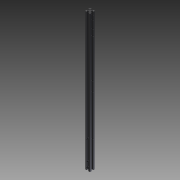
# Autodesk Inventor part: HFSB5-2020-550-LCH-RWV-AH30-BH60-CH85-DH240-EH280-AP442
Saved by Autodesk Inventor 2011 SP1 (Build 150282100, 282)
## iProperties
Created: 2016-03-22
Part Number: HFSB5-2020-550-LCH-RWV-AH30-BH60-CH85-DH240-EH280-AP442
Catalog Web Link: www.cadenas.de
Description: NFS5-2020, NFSB5-2020, HFS5-2020, HFSB5-2020, CAF5-2020, HFSY5-2020, NFSF5-2020, HFSF5-2020, HFSFB5-2020, NFST5-2020, HFST5-2020, HFSTB5-2020, HFSH5-2020, HFSC5-2020-HFS5 Series Aluminum Extrusions 20 Square -1 Slot-
Vendor: MISUMI
Document SubType Name: Modeling
Designer: psAdmin
Manufacturer: MISUMI
Mass: 97.771 g
Surface Area: 953.438 cm^2
Volume: 97.771 cm^3
Density: 1 g/cm^3
Category: PARTsolutions
Company: MISUMI
Title: HFSB5-2020-550-LCH-RWV-AH30-BH60-CH85-DH240-EH280-AP442
Author: Cadenas PARTsolutions
Comments: HFS5 Series Aluminum Extrusions 20 Square -1 Slot-
PSOL_IDENT_0: {$CADENAS_DATA\23d-libs\misumi\metric\38_al_extrusions_blackets\5\hfs5_2020.prj},654 {VTYP=3D},{NB=H
PSOL_IDENT_1: FSB5-2020-550-LCH-RWV-AH30-BH60-CH85-DH240-EH280-AP442},{LINA=HFSB5-2020-550-LCH-RWV-AH30-BH60-CH85-
PSOL_IDENT_2: DH240-EH280-AP442},{NN=NFS5-2020, NFSB5-2020, HFS5-2020, HFSB5-2020, CAF5-2020, HFSY5-2020, NFSF5-20
PSOL_IDENT_3: 20, HFSF5-2020, HFSFB5-2020, NFST5-2020, HFST5-2020, HFSTB5-2020, HFSH5-2020, HFSC5-2020},{DATE=17.0
PSOL_IDENT_4: 7.2015 10:47:07},{GEOMDATE=28.10.2014 00:00:00},{VERSION=},{LINEID=140},{LINESUBID=-1},{WBVAR=L,ALT1
PSOL_IDENT_5: ,ALT2,ALT4,ALT5,CP5,DL5,DR5,ALT6,ALT9,ALT10,ALT11,HP6,NHL6,DL6,NHR6,DR6,ALT7,ALT8,NH9,AH,BH,CH,DH,EH
PSOL_IDENT_6: ,NH10,AV,BV,CV,DV,EV,NH11,AP,BP,CP,DP,EP,ALT12,ALT13,Z,NH12,XA,XB,XC,XD,XE,NH13,YA,YB,YC,YD,YE,ALT16
PSOL_IDENT_7: ,HP16,DL16,DR16,ALT17,HQ17,JLP,ALT20}  {NB=HFSB5-2020-550-LCH-RWV-AH30-BH60-CH85-DH240-EH280-AP442},
PSOL_IDENT_8: {LINA=HFSB5-2020-550-LCH-RWV-AH30-BH60-CH85-DH240-EH280-AP442},{KT=DUMMY},{PN=HFSB5-2020-550-LCH-RWV
PSOL_IDENT_9: -AH30-BH60-CH85-DH240-EH280-AP442},{TPS=HFSB5-2020},{MAT=A6N01SS-T5 Aluminum Alloy or 6005A-T5 Alumi
PSOL_IDENT_10: num Alloy},{ST=Black Anodize},{FRMW=20},{FRMH=20},{FRD=4.2},{L=550},{MASS=0.5},{SA=183},{LX=0.742x10
PSOL_IDENT_11: ^4},{LY=0.742x10^4},{ALT1=},{M1=0},{DPL1=0},{DPR1=0},{ALT1PN=},{ALT2=},{ALT2ALG= '','w/o End Tapping
PSOL_IDENT_12: (Heli-Coil Insert)','LHP','with LHP (Tapping on the Left (Heli-Coil Insert))','RHP','with RHP (Tapp
PSOL_IDENT_13: ing on the Right (Heli-Coil Insert))','HPW','with HPW (Tapping on Both Ends (Heli-Coil Insert))' },{
PSOL_IDENT_14: M2=0},{DP2=0},{ALT2PN=},{ALT4=},{ALT4ALG= '', 'w/o SC (High Precision Cut)', 'SC', 'with SC (High Pr
PSOL_IDENT_15: ecision Cut)' },{ALT4PN=},{ALT5=},{ALT5ALG= '','w/o 45 Degree Cut','1','with 45 Degree Cut' },{CP5=}
PSOL_IDENT_16: ,{CP5ALG= '','N/A' },{DL5=},{DL5ALG= '','N/A' },{DR5=},{DR5ALG= '','N/A' },{FRMLALT5=0},{FRMRALT5=0}
PSOL_IDENT_17: ,{ALT5PN=},{ALT6=1},{ALT6ALG= '','w/o Fastening Location Wrench Access Hole Alterations','1','with F
PSOL_IDENT_18: astening Location Wrench Access Hole Alterations' },{ALT9=1},{ALT9ALG= '','w/o Location Specified Wr
PSOL_IDENT_19: ench Access Hole Alteratons (Horizontal)','1','with Location Specified Wrench Access Hole Alteratons
PSOL_IDENT_20: (Horizontal)' },{ALT10=},{ALT10ALG= '','w/o Location Specified Wrench Access Hole Alteratons (Verti
PSOL_IDENT_21: cal)','1','with Location Specified Wrench Access Hole Alteratons (Vertical)' },{ALT11=1},{ALT11ALG= ''
PSOL_IDENT_22: ,'w/o Location Specified Wrench Access Hole Alteratons (Crisscross)','1','with Location Specified Wr
PSOL_IDENT_23: ench Access Hole Alteratons (Crisscross)' },{HP6=LR},{HP6ALG= 'L','Left','R','Right','LR','Both Side
PSOL_IDENT_24: s' },{NHL6=C},{NHL6ALG= 'C','C (Wrench Holes in Single Line)','W','W (Wrench Holes in Two Lines)','E'
PSOL_IDENT_25: ,'E (Wrench Holes in Three Lines)' },{DL6=H},{DL6ALG= 'H','H (Horizontal)','V','V (Vertical)','P','P
PSOL_IDENT_26: (Crisscross)' },{NHR6=W},{NHR6ALG= 'C','C (Wrench Holes in Single Line)','W','W (Wrench Holes in Tw
PSOL_IDENT_27: o Lines)','E','E (Wrench Holes in Three Lines)' },{DR6=V},{DR6ALG= 'H','H (Horizontal)','V','V (Vert
PSOL_IDENT_28: ical)','P','P (Crisscross)' },{HL6=10},{HL6D=10},{HR6=10},{HR6D=10},{J6=20},{J6D=20},{K6=20},{K6D=0}
PSOL_IDENT_29: ,{DD6=7.35},{DD6ALG=7.35},{ALT7=},{ALT7ALG= '','w/o FL (Shifts The Wrench Hole on The Left Side 3mm
PSOL_IDENT_30: Toward The Left End)','FL','with FL (Shifts The Wrench Hole on The Left Side 3mm Toward The Left End
PSOL_IDENT_31: )' },{ALT8=},{ALT8ALG= '','w/o FR (Shifts The Wrench Hole on The Right Side 3mm Toward The Right End
PSOL_IDENT_32: )','FR','with FR (Shifts The Wrench Hole on The Right Side 3mm Toward The Right End)' },{ALT678PN=-L
PSOL_IDENT_33: CH-RWV},{NH9=5},{NH9MAX=5},{NH9ALG=[1:5/1]},{AH=30.0},{AHMIN=7},{AHMAX=505},{AHALG=[7:505/0.5]},{BH=
PSOL_IDENT_34: 60.0},{BHMIN=39.5},{BHMAX=514.5},{BHALG=[39.5:514.5/0.5]},{CH=85.0},{CHMIN=69.5},{CHMAX=524},{CHALG=
PSOL_IDENT_35: [69.5:524/0.5]},{DH=240.0},{DHMIN=94.5},{DHMAX=533.5},{DHALG=[94.5:533.5/0.5]},{EH=280.0},{EHMIN=249
PSOL_IDENT_36: .5},{EHMAX=543},{EHALG=[249.5:543/0.5]},{NH10=0},{NH10MAX=5},{NH10ALG=[0]},{AV=0.0},{AVMIN=7},{AVMAX=
PSOL_IDENT_37: 552.5},{AVALG=[0]},{BV=0.0},{BVMIN=9.5},{BVMAX=562},{BVALG=[0]},{CV=0.0},{CVMIN=9.5},{CVMAX=571.5},{
PSOL_IDENT_38: CVALG=[0]},{DV=0.0},{DVMIN=9.5},{DVMAX=581},{DVALG=[0]},{EV=0.0},{EVMIN=9.5},{EVMAX=543},{EVALG=[0]}
PSOL_IDENT_39: ,{NH11=1},{NH11MAX=5},{NH11ALG=[1:5/1]},{AP=442.0},{APMIN=7},{APMAX=543},{APALG=[7:543/0.5]},{BP=0.0
PSOL_IDENT_40: },{BPMIN=451.5},{BPMAX=552.5},{BPALG=[0]},{CP=0.0},{CPMIN=9.5},{CPMAX=562},{CPALG=[0]},{DP=0.0},{DPM
PSOL_IDENT_41: IN=9.5},{DPMAX=571.5},{DPALG=[0]},{EP=0.0},{EPMIN=9.5},{EPMAX=543},{EPALG=[0]},{ALT9PN=-AH30-BH60-CH
PSOL_IDENT_42: 85-DH240-EH280},{ALT10PN=},{ALT11PN=-AP442},{ALT91011PN=-AH30-BH60-CH85-DH240-EH280-AP442},{ALT12=},
PSOL_IDENT_43: {ALT12ALG= '','w/o Counterbore Hole in Specified Position (Vertical)','1','with Counterbore Hole in
PSOL_IDENT_44: Specified Position (Vertical)' },{ALT13=},{ALT13ALG= '','w/o Counterbore Hole in Specified Position
PSOL_IDENT_45: (Horizontal)','1','with Counterbore Hole in Specified Position (Horizontal)' },{Z=},{ZALG= '','N/A'
PSOL_IDENT_46: },{DD12=0.0},{DD112=0.0},{NH12=0},{NH12MAX=5},{NH12ALG=[0]},{XA=0.0},{XAMIN=7},{XAMAX=545},{XAALG=[0
PSOL_IDENT_47: ]},{XB=0.0},{XBMIN=2},{XBMAX=547},{XBALG=[0]},{XC=0.0},{XCMIN=2},{XCMAX=549},{XCALG=[0]},{XD=0.0},{X
PSOL_IDENT_48: DMIN=2},{XDMAX=551},{XDALG=[0]},{XE=0.0},{XEMIN=2},{XEMAX=543},{XEALG=[0]},{NH13=0},{NH13MAX=5},{NH1
PSOL_IDENT_49: 3ALG=[0]},{YA=0.0},{YAMIN=7},{YAMAX=545},{YAALG=[0]},{YB=0.0},{YBMIN=2},{YBMAX=547},{YBALG=[0]},{YC=
PSOL_IDENT_50: 0.0},{YCMIN=2},{YCMAX=549},{YCALG=[0]},{YD=0.0},{YDMIN=2},{YDMAX=551},{YDALG=[0]},{YE=0.0},{YEMIN=2}
PSOL_IDENT_51: ,{YEMAX=543},{YEALG=[0]},{ALT12PN=},{ALT13PN=},{ALT1213PN=},{ALT16=},{ALT16ALG= '','w/o M Type Hole
PSOL_IDENT_52: Alteration','1','with M Type Hole Alteration' },{HP16=},{HP16ALG= '','N/A' },{DL16=},{DL16ALG= '','N
PSOL_IDENT_53: /A' },{DR16=},{DR16ALG= '','N/A' },{H116=0},{D16=0.0},{ALT16PN=},{ALT17=},{ALT17ALG= '','w/o L Type
PSOL_IDENT_54: Hole Alteration (Top)','1','with L Type Hole Alteration (Top)' },{HQ17=0},{HQ17ALG=0},{JLP=0},{JLPMI
PSOL_IDENT_55: N=4.9},{JLPMAX=0},{JLPALG=[0]},{L17=0},{D17=0.0},{ALT17PN=},{ALT20=},{ALT20PN=},{ERRORALT01=OK},{ERR
PSOL_IDENT_56: ORALT02=OK},{ERRORALT05=OK},{ERRORALT06091=OK},{ERRORALT06092=OK},{ERRORALT06093=OK},{ERRORALT06094=
PSOL_IDENT_57: OK},{ERRORALT06101=OK},{ERRORALT06102=OK},{ERRORALT06103=OK},{ERRORALT06104=OK},{ERRORALT06111=OK},{
PSOL_IDENT_58: ERRORALT06112=OK},{ERRORALT06113=OK},{ERRORALT06114=OK},{ERRORALT06121=OK},{ERRORALT06122=OK},{ERROR
PSOL_IDENT_59: ALT06123=OK},{ERRORALT06124=OK},{ERRORALT06131=OK},{ERRORALT06132=OK},{ERRORALT06133=OK},{ERRORALT06
PSOL_IDENT_60: 134=OK},{ERRORALT0616=OK},{ERRORALT06171=OK},{ERRORALT06172=OK},{ERRORALT06173=OK},{ERRORALT0911=OK}
PSOL_IDENT_61: ,{ERRORALT0913=OK},{ERRORALT0916=OK},{ERRORALT0917=OK},{ERRORALT1011=OK},{ERRORALT1012=OK},{ERRORALT
PSOL_IDENT_62: 1016=OK},{ERRORALT1017=OK},{ERRORALT1112=OK},{ERRORALT1113=OK},{ERRORALT1116=OK},{ERRORALT1117=OK},{
PSOL_IDENT_63: ERRORALT1216=OK},{ERRORALT1217=OK},{ERRORALT1316=OK},{ERRORALT1317=OK},{ERRORALT1617=OK},{ERRORPN=},
PSOL_IDENT_64: {TFW=0}
NN: NFS5-2020, NFSB5-2020, HFS5-2020, HFSB5-2020, CAF5-2020, HFSY5-2020, NFSF5-2020, HFSF5-2020, HFSFB5-2020, NFST5-2020, HFST5-2020, HFSTB5-2020, HFSH5-2020, HFSC5-2020
NT: HFS5 Series Aluminum Extrusions 20 Square -1 Slot-
NB: HFSB5-2020-550-LCH-RWV-AH30-BH60-CH85-DH240-EH280-AP442
NBSYN: $PN.
LINA: HFSB5-2020-550-LCH-RWV-AH30-BH60-CH85-DH240-EH280-AP442
PN: HFSB5-2020-550-LCH-RWV-AH30-BH60-CH85-DH240-EH280-AP442
TPS: HFSB5-2020
MAT: A6N01SS-T5 Aluminum Alloy or 6005A-T5 Aluminum Alloy
ST: Black Anodize
L: 550
MASS: 0.5
SA: 183
LX: 0.742x10^4
LY: 0.742x10^4
ALT1: w/o End Tapping
M1: 0
DPL1: 0
DPR1: 0
ALT2: w/o End Tapping (Heli-Coil Insert)
M2: 0
DP2: 0
ALT4: w/o SC (High Precision Cut)
ALT5: w/o 45 Degree Cut
CP5: N/A
DL5: N/A
DR5: N/A
ALT6: with Fastening Location Wrench Access Hole Alterations
ALT9: with Location Specified Wrench Access Hole Alteratons (Horizontal)
ALT10: w/o Location Specified Wrench Access Hole Alteratons (Vertical)
ALT11: with Location Specified Wrench Access Hole Alteratons (Crisscross)
HP6: Both Sides
NHL6: C (Wrench Holes in Single Line)
DL6: H (Horizontal)
NHR6: W (Wrench Holes in Two Lines)
DR6: V (Vertical)
HL6D: 10
HR6D: 10
J6D: 20
K6D: 0
DD6: 7.35
ALT7: w/o FL (Shifts The Wrench Hole on The Left Side 3mm Toward The Left End)
ALT8: w/o FR (Shifts The Wrench Hole on The Right Side 3mm Toward The Right End)
NH9: 5
AH: 30.0
BH: 60.0
CH: 85.0
DH: 240.0
EH: 280.0
NH10: 0
AV: 0.0
BV: 0.0
CV: 0.0
DV: 0.0
EV: 0.0
NH11: 1
AP: 442.0
BP: 0.0
CP: 0.0
DP: 0.0
EP: 0.0
ALT12: w/o Counterbore Hole in Specified Position (Vertical)
ALT13: w/o Counterbore Hole in Specified Position (Horizontal)
Z: N/A
DD12: 0.0
DD112: 0.0
NH12: 0
XA: 0.0
XB: 0.0
XC: 0.0
XD: 0.0
XE: 0.0
NH13: 0
YA: 0.0
YB: 0.0
YC: 0.0
YD: 0.0
YE: 0.0
ALT16: w/o M Type Hole Alteration
HP16: N/A
DL16: N/A
DR16: N/A
H116: 0
D16: 0.0
ALT17: w/o L Type Hole Alteration (Top)
HQ17: 0
JLP: 0
D17: 0.0
ALT20: w/o CW (End Face C Chamfering)
SUPPLIER: MISUMI
ARTICLENO: HFSB5-2020-550-LCH-RWV-AH30-BH60-CH85-DH240-EH280-AP442
BOMINFO: HFSB5-2020-550-LCH-RWV-AH30-BH60-CH85-DH240-EH280-AP442
CREATOR: CADENAS GmbH
Autodesk Inventor part; units mm, degrees
ref_plane "YZ Plane" through (0, 0, 0) normal (1, 0, 0) x (0, 1, 0)
ref_plane "XZ Plane" through (0, 0, 0) normal (0, 1, 0) x (-1, 0, 0)
ref_plane "XY Plane" through (0, 0, 0) normal (0, 0, 1) x (1, 0, 0)
sketch "Sketch_1" plane through (0, 0, 0) normal (0, 0, 1) x (1, 0, 0)
  line L0 (-10, 3) -> (-8, 3)
  line L1 (-8, 3) -> (-8, 6)
  line L2 (-8, 6) -> (-7.0607, 6)
  line L3 (-7.0607, 6) -> (-4, 2.9393)
  line L4 (-4, 2.9393) -> (-4, 0.5196)
  line L5 (-4, 0.5196) -> (-3.7, 0)
  line L6 (-3.7, 0) -> (-4, -0.5196)
  line L7 (-4, -0.5196) -> (-4, -2.9393)
  line L8 (-4, -2.9393) -> (-7.0607, -6)
  line L9 (-7.0607, -6) -> (-8, -6)
  line L10 (-8, -6) -> (-8, -3)
  line L11 (-8, -3) -> (-10, -3)
  line L12 (-10, -3) -> (-10, -9)
  arc A0 (-10, -9) -> (-9, -10) centre (-9, -9) ccw
  line L13 (-9, -10) -> (-3, -10)
  line L14 (-3, -10) -> (-3, -8)
  line L15 (-3, -8) -> (-6, -8)
  line L16 (-6, -8) -> (-6, -7.0607)
  line L17 (-6, -7.0607) -> (-2.9393, -4)
  line L18 (-2.9393, -4) -> (-0.5196, -4)
  line L19 (-0.5196, -4) -> (0, -3.7)
  line L20 (0, -3.7) -> (0.5196, -4)
  line L21 (0.5196, -4) -> (2.9393, -4)
  line L22 (2.9393, -4) -> (6, -7.0607)
  line L23 (6, -7.0607) -> (6, -8)
  line L24 (6, -8) -> (3, -8)
  line L25 (3, -8) -> (3, -10)
  line L26 (3, -10) -> (9, -10)
  arc A1 (9, -10) -> (10, -9) centre (9, -9) ccw
  line L27 (10, -9) -> (10, -3)
  line L28 (10, -3) -> (8, -3)
  line L29 (8, -3) -> (8, -6)
  line L30 (8, -6) -> (7.0607, -6)
  line L31 (7.0607, -6) -> (4, -2.9393)
  line L32 (4, -2.9393) -> (4, -0.5196)
  line L33 (4, -0.5196) -> (3.7, 0)
  line L34 (3.7, 0) -> (4, 0.5196)
  line L35 (4, 0.5196) -> (4, 2.9393)
  line L36 (4, 2.9393) -> (7.0607, 6)
  line L37 (7.0607, 6) -> (8, 6)
  line L38 (8, 6) -> (8, 3)
  line L39 (8, 3) -> (10, 3)
  line L40 (10, 3) -> (10, 9)
  arc A2 (10, 9) -> (9, 10) centre (9, 9) ccw
  line L41 (9, 10) -> (3, 10)
  line L42 (3, 10) -> (3, 8)
  line L43 (3, 8) -> (6, 8)
  line L44 (6, 8) -> (6, 7.0607)
  line L45 (6, 7.0607) -> (2.9393, 4)
  line L46 (2.9393, 4) -> (0.5196, 4)
  line L47 (0.5196, 4) -> (0, 3.7)
  line L48 (0, 3.7) -> (-0.5196, 4)
  line L49 (-0.5196, 4) -> (-2.9393, 4)
  line L50 (-2.9393, 4) -> (-6, 7.0607)
  line L51 (-6, 7.0607) -> (-6, 8)
  line L52 (-6, 8) -> (-3, 8)
  line L53 (-3, 8) -> (-3, 10)
  line L54 (-3, 10) -> (-9, 10)
  arc A3 (-9, 10) -> (-10, 9) centre (-9, 9) ccw
  line L55 (-10, 9) -> (-10, 3)
  constraints: 112 end point, 8 point on circle, 4 centre point
extrude "Extrusion1" add sketch "Sketch_1" against normal blind 550
sketch "Sketch2" plane through (0, 0, -550) normal (0, 0, -1) x (-1, 0, 0)
  point P0 (0, 0)
hole "Hole1" at (0, 0, -550) direction (0, 0, 1) diameter 4.2 depth 550
sketch "Sketch_13" plane through (0, 0, 0) normal (0, 1, 0) x (1, 0, 0)
  line L0 (10, 10) -> (-10, 10)
  line L1 (-10, 10) -> (-10, 13.675)
  line L2 (-10, 13.675) -> (10, 13.675)
  line L3 (10, 13.675) -> (10, 10)
  line L4 (10, 10) -> (-10, 10)
  constraints: 10 end point
revolve "Revolution1" cut sketch "Sketch_13" angle 360 about axis through (10, 0, -10) along (1, 0, 0)
sketch "Sketch_22" plane through (0, 0, 0) normal (1, 0, 0) x (0, 0, -1)
  line L0 (540, -10) -> (540, 10)
  line L1 (540, 10) -> (543.675, 10)
  line L2 (543.675, 10) -> (543.675, -10)
  line L3 (543.675, -10) -> (540, -10)
  line L4 (540, -10) -> (540, 10)
  constraints: 10 end point
revolve "Revolution2" cut sketch "Sketch_22" angle 360 about axis through (0, -10, -540) along (0, -1, 0)
sketch "Sketch_23" plane through (0, 0, 0) normal (1, 0, 0) x (0, 0, -1)
  line L0 (520, -10) -> (520, 10)
  line L1 (520, 10) -> (523.675, 10)
  line L2 (523.675, 10) -> (523.675, -10)
  line L3 (523.675, -10) -> (520, -10)
  line L4 (520, -10) -> (520, 10)
  constraints: 10 end point
revolve "Revolution3" cut sketch "Sketch_23" angle 360 about axis through (0, -10, -520) along (0, -1, 0)
sketch "Sketch_62" plane through (0, 0, 0) normal (0, 1, 0) x (1, 0, 0)
  line L0 (10, 30) -> (-10, 30)
  line L1 (-10, 30) -> (-10, 33.675)
  line L2 (-10, 33.675) -> (10, 33.675)
  line L3 (10, 33.675) -> (10, 30)
  line L4 (10, 30) -> (-10, 30)
  constraints: 10 end point
revolve "Revolution4" cut sketch "Sketch_62" angle 360 about axis through (10, 0, -30) along (1, 0, 0)
sketch "Sketch_25" plane through (0, 0, 0) normal (0, 1, 0) x (1, 0, 0)
  line L0 (10, 60) -> (-10, 60)
  line L1 (-10, 60) -> (-10, 63.675)
  line L2 (-10, 63.675) -> (10, 63.675)
  line L3 (10, 63.675) -> (10, 60)
  line L4 (10, 60) -> (-10, 60)
  constraints: 10 end point
revolve "Revolution5" cut sketch "Sketch_25" angle 360 about axis through (10, 0, -60) along (1, 0, 0)
sketch "Sketch_26" plane through (0, 0, 0) normal (0, 1, 0) x (1, 0, 0)
  line L0 (10, 85) -> (-10, 85)
  line L1 (-10, 85) -> (-10, 88.675)
  line L2 (-10, 88.675) -> (10, 88.675)
  line L3 (10, 88.675) -> (10, 85)
  line L4 (10, 85) -> (-10, 85)
  constraints: 10 end point
revolve "Revolution6" cut sketch "Sketch_26" angle 360 about axis through (10, 0, -85) along (1, 0, 0)
sketch "Sketch_27" plane through (0, 0, 0) normal (0, 1, 0) x (1, 0, 0)
  line L0 (10, 240) -> (-10, 240)
  line L1 (-10, 240) -> (-10, 243.675)
  line L2 (-10, 243.675) -> (10, 243.675)
  line L3 (10, 243.675) -> (10, 240)
  line L4 (10, 240) -> (-10, 240)
  constraints: 10 end point
revolve "Revolution7" cut sketch "Sketch_27" angle 360 about axis through (10, 0, -240) along (1, 0, 0)
sketch "Sketch_28" plane through (0, 0, 0) normal (0, 1, 0) x (1, 0, 0)
  line L0 (10, 280) -> (-10, 280)
  line L1 (-10, 280) -> (-10, 283.675)
  line L2 (-10, 283.675) -> (10, 283.675)
  line L3 (10, 283.675) -> (10, 280)
  line L4 (10, 280) -> (-10, 280)
  constraints: 10 end point
revolve "Revolution8" cut sketch "Sketch_28" angle 360 about axis through (10, 0, -280) along (1, 0, 0)
sketch "Sketch_36" plane through (0, 0, 0) normal (0, 1, 0) x (1, 0, 0)
  line L0 (10, 442) -> (-10, 442)
  line L1 (-10, 442) -> (-10, 445.675)
  line L2 (-10, 445.675) -> (10, 445.675)
  line L3 (10, 445.675) -> (10, 442)
  line L4 (10, 442) -> (-10, 442)
  constraints: 10 end point
revolve "Revolution9" cut sketch "Sketch_36" angle 360 about axis through (10, 0, -442) along (1, 0, 0)
sketch "Sketch_37" plane through (0, 0, 0) normal (1, 0, 0) x (0, 0, -1)
  line L0 (442, -10) -> (442, 10)
  line L1 (442, 10) -> (445.675, 10)
  line L2 (445.675, 10) -> (445.675, -10)
  line L3 (445.675, -10) -> (442, -10)
  line L4 (442, -10) -> (442, 10)
  constraints: 10 end point
revolve "Revolution10" cut sketch "Sketch_37" angle 360 about axis through (0, -10, -442) along (0, -1, 0)
ref_plane "C1_XY" through (0, 0, 0) normal (0, 0, 1) x (1, 0, 0)
ref_plane "C1_YZ" through (0, 0, 0) normal (1, 0, 0) x (0, 1, 0)
ref_plane "C1_ZX" through (0, 0, 0) normal (0, 1, 0) x (0, 0, 1)
body "Solid1"
